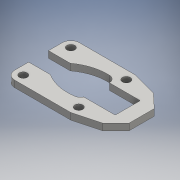
# Autodesk Inventor part: 스케치02
Saved by Autodesk Inventor 2016 (Build 200138000, 138)
## iProperties
Created: 2024-04-19
Part Number: 스케치02
Material: 일반
Document SubType Name: Modeling
Designer: pc
Density: 1 g/cm^3
Appearance: 기본값
Author: pc
Autodesk Inventor part; units mm, degrees
ref_plane "YZ Plane" through (0, 0, 0) normal (1, 0, 0) x (0, 1, 0)
ref_plane "XZ Plane" through (0, 0, 0) normal (0, 1, 0) x (-1, 0, 0)
ref_plane "XY Plane" through (0, 0, 0) normal (0, 0, 1) x (1, 0, 0)
sketch "스케치1" plane through (0, 0, 0) normal (0, 0, 1) x (1, 0, 0)
  line L0 (-26.6915, 0) -> (30.6457, 0)
  line L1 (0.0002, 26.0752) -> (0.0002, -24.1528)
  line L2 (-65.2443, -49.1703) -> (0.0002, -49.1703)
  line L3 (0.0002, 48.8297) -> (-65.2443, 48.8297)
  line L4 (-78.2443, -49.1703) -> (77.7557, 48.8632) construction
  line L5 (78.0463, -48.7061) -> (-78.2443, 48.8297) construction
  line L6 (-65.2443, 35.8297) -> (18.7557, 35.8297)
  line L7 (18.7557, 35.8297) -> (18.7557, -36.1703)
  line L8 (18.7557, -36.1703) -> (-65.2443, -36.1703)
  line L9 (-65.2443, -36.1703) -> (-65.2443, 35.8297)
  line L10 (56.7557, 17.5022) -> (56.7557, -17.4978)
  circle A0 centre (18.7557, 35.8297) radius 6
  circle A1 centre (-65.2443, 35.8297) radius 6
  circle A2 centre (18.7557, -36.1703) radius 6
  circle A3 centre (-65.2443, -36.1703) radius 6
  arc A4 (-65.2443, 48.8297) -> (-78.2443, 35.8297) centre (-65.2443, 35.8297) ccw
  arc A5 (-78.2443, -36.1703) -> (-65.2443, -49.1703) centre (-65.2443, -36.1703) ccw
  line L11 (77.7557, -19) -> (77.7557, 19)
  line L12 (0.0002, 48.8297) -> (82.2012, 48.8297) construction
  line L13 (-78.2443, -49.1703) -> (82.2012, -49.1703) construction
  line L14 (0.0002, -49.1703) -> (19.6899, -49.1703)
  line L15 (0.0002, 48.8297) -> (19.0402, 48.8297)
  line L16 (19.6899, -49.1703) -> (57.7958, -38.9598)
  line L17 (19.6899, -49.1703) -> (59.1401, -49.1703) construction
  line L18 (19.0402, 48.8297) -> (59.7283, 48.8297) construction
  line L19 (57.7958, -38.9598) -> (87.4943, -38.9598) construction
  line L20 (19.0402, 48.8297) -> (61.8181, 48.8297) construction
  line L21 (19.0402, 48.8297) -> (57.0006, 38.6583)
  line L22 (19.0402, 48.8297) -> (58.3397, 48.8297) construction
  line L23 (57.0006, 38.6583) -> (77.7557, 19)
  line L24 (57.7958, -38.9598) -> (77.7557, -19)
  arc A6 (10.0002, 19.0022) -> (-0.0006, 29.0001) centre (0.0002, 19.0001) ccw
  line L25 (-78.2443, 35.8297) -> (-78.2443, 15.0001)
  line L26 (-78.2443, -15.0002) -> (-78.2443, -36.1703)
  line L27 (10.0002, 19.0022) -> (55.2557, 19.0022)
  line L28 (55.2557, -18.9978) -> (9.1632, -18.9978)
  line L29 (-45.2992, -15.0002) -> (-78.2443, -15.0002)
  arc A7 (-45.2992, -15.0002) -> (-0.0006, -24.9934) centre (-9.1955, 40.9912) ccw
  arc A8 (-0.0006, 29.0001) -> (-45.2992, 15.0001) centre (-2.8258, -42.143) ccw
  arc A9 (-0.0006, -24.9934) -> (9.1632, -18.9978) centre (0.0002, -14.9938) ccw
  arc A10 (56.7557, 17.5022) -> (55.2557, 19.0022) centre (55.2557, 17.5022) ccw
  arc A11 (55.2557, -18.9978) -> (56.7557, -17.4978) centre (55.2557, -17.4978) ccw
  line L30 (-78.2443, 15.0001) -> (-45.2992, 15.0001)
  point P0 (0, 0)
  dimension "d0" = 156
  dimension "d1" = 98
  dimension "d2" = 13
  dimension "d4" = 13
  dimension "d5" = 84
  dimension "d6" = 38
  dimension "d8" = 12
  dimension "d9" = 12
  dimension "d10" = 12
  dimension "d11" = 12
  dimension "d12" = 13
  dimension "d15" = 38
  dimension "d17" = 15
  dimension "d21" = 15
  dimension "d23" = 45
  dimension "d27" = 20
  dimension "d29" = 3
  dimension "d30" = 3
  dimension "d31" = 30.0004
  constraints: 62 end point, 16 point on circle, 13 horizontal, 12 centre point, 12 point on line, 10 tangent, 7 parallel, 4 coincident, 3 perpendicular, 2 equal length, 1 equal radius, 1 vertical
  measures "d0" distance of L5.end L4.end
  measures "d1" distance of L4.start L5.end
  measures "d2" distance between parallel lines of L2 L8
  measures "d4" distance between parallel lines of L3 L6
  measures "d5" distance of L7.end L8.end
  measures "d6" distance of L27.end L28.start
  measures "d8" diameter of A0
  measures "d9" diameter of A1
  measures "d10" diameter of A2
  measures "d11" diameter of A3
  measures "d12" radius of A4
  measures "d15" distance from line of L10 L7.end
  measures "d17" angle of L17 L16
  measures "d21" angle of L21 L22
  measures "d23" angle of L11 L24
  measures "d27" diameter of A6
  measures "d29" diameter of A10
  measures "d30" diameter of A11
  measures "d31" distance between parallel lines of L29 L30
extrude "돌출1" add sketch "스케치1" along normal blind 10 contours A5 L26 L29 L9 A3 L8 A2 L7 L28 A11 L10 A10 L27 A0 L6 A1 L30 L25 A4 L3 L15 L21 L23 L11 L24 L16 L14 L2 | L29 A7 A9 L28 L7 A2 L8 A3 L9 | L9 A1 L6 A0 L7 L27 A6 A8 L30
